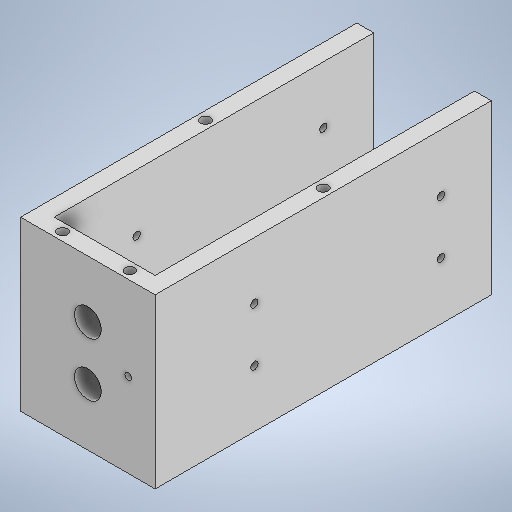
# Autodesk Inventor part: Handle_Main_Body
Saved by Autodesk Inventor 2026.2 (Build 302298010, 298A)
## iProperties
Created: 2026-04-30
Part Number: Handle_Main_Body
Material: Generic
Document SubType Name: Modeling
Designer: piete
Density: 1 g/cm^3
Appearance: Default
Author: piete
Autodesk Inventor part; units mm, degrees
ref_plane "YZ Plane" through (0, 0, 0) normal (1, 0, 0) x (0, 1, 0)
ref_plane "XY Plane" through (0, 0, 0) normal (0, 0, 1) x (1, 0, 0)
sketch "Sketch1" plane through (0, 0, 0) normal (0, 1, 0) x (-1, 0, 0)
  line L0 (20, 50) -> (-20, 50)
  line L1 (-20, 50) -> (-20, -50)
  line L2 (-20, -50) -> (20, -50)
  line L3 (20, -50) -> (20, 50)
  line L4 (15, 45) -> (-15, 45)
  line L5 (-15, 45) -> (-15, -45)
  line L6 (-15, -45) -> (15, -45)
  line L7 (15, -45) -> (15, 45)
  line L8 (15, -45) -> (15, -50)
  line L9 (-15, -45) -> (-15, -50)
  point P0 (0, 0)
  dimension "d0" = 40
  dimension "d1" = 100
  dimension "d2" = 20
  dimension "d3" = 50
  dimension "d4" = 5
  constraints: 20 end point, 4 parallel, 4 perpendicular, 2 point on line, 1 horizontal, 3 other
  measures "d0" distance of L2.end L1.end
  measures "d1" distance of L1.end L0.end
  measures "d2" distance from line of point (0, 0) L3
  measures "d3" distance from line of point (0, 0) L0
  measures "d4" distance between parallel lines of L3 L7
extrude "Extrusion1" add sketch "Sketch1" along normal blind 50 contours L3 L2 L8 L7 L4 L5 L9 L1 L0
sketch "Sketch2" plane through (-20, 0, 50) normal (0, 0, 1) x (1, 0, 0)
  circle A0 centre (20, 33) radius 4
  circle A1 centre (20, 17) radius 4
  circle A2 centre (32, 25) radius 1
  line L0 (0, 0) -> (40, 0) projected
  line L1 (40, 0) -> (40, 50) projected
  point P0 (20, 0)
  point P1 (20, 0)
  point P2 (20, 0)
  dimension "d7" = 8
  dimension "d8" = 8
  dimension "d9" = 2
  dimension "d10" = 0
  dimension "d11" = 0
  dimension "d12" = 8
  dimension "d13" = 25
  dimension "d14" = 16
  dimension "d15" = 8
  constraints: 3 centre point, 2 midpoint
  measures "d7" diameter of A0
  measures "d8" diameter of A1
  measures "d9" diameter of A2
  measures "d10" horizontal distance of point (20, 0) A0.centre
  measures "d11" horizontal distance of point (20, 0) A1.centre
  measures "d12" distance from line of L1 A2.centre
  measures "d13" distance from line of L0 A2.centre
  measures "d14" distance of A0.centre A1.centre
  measures "d15" vertical distance of A1.centre A2.centre
extrude "Extrusion2" cut sketch "Sketch2" against normal up to surface (5 mm away)
sketch "Sketch3" plane through (-20, 0, 50) normal (0, 0, 1) x (1, 0, 0)
  circle A0 centre (20, 33) radius 4 projected
  circle A1 centre (20, 33) radius 6
  circle A2 centre (20, 17) radius 4 projected
  circle A3 centre (20, 17) radius 6
  point P0 (20, 0)
  dimension "d18" = 12
  dimension "d19" = 12
  constraints: 2 centre point, 2 coincident
  measures "d18" diameter of A1
  measures "d19" diameter of A3
extrude "Extrusion3" add sketch "Sketch3" against normal blind 8
sketch "Sketch4" plane through (-15, 0, -50) normal (0, 0, -1) x (-1, 0, 0)
  circle A0 centre (2.5, 47.5) radius 1.5
  line L0 (5, 0) -> (5, 50) projected
  line L1 (0, 50) -> (5, 50) projected
  circle A1 centre (-32.5, 47.5) radius 1.5
  line L2 (-35, 50) -> (-30, 50) projected
  line L3 (-35, 0) -> (-35, 50) projected
  circle A2 centre (-32.5, 2.5) radius 1.5
  circle A3 centre (2.5, 2.5) radius 1.5
  line L4 (-35, 0) -> (-30, 0) projected
  line L5 (0, 0) -> (5, 0) projected
  point P0 (-15, 0)
  point P1 (-32.5, 50)
  dimension "d22" = 3
  dimension "d23" = 2.5
  dimension "d24" = 2.5
  dimension "d25" = 3
  dimension "d26" = 2.5
  dimension "d27" = 2.5
  dimension "d28" = 3
  dimension "d29" = 3
  dimension "d30" = 2.5
  dimension "d31" = 2.5
  dimension "d32" = 2.5
  dimension "d33" = 2.5
  constraints: 4 centre point, 1 midpoint
  measures "d22" diameter of A0
  measures "d23" distance from line of L0 A0.centre
  measures "d24" distance from line of L1 A0.centre
  measures "d25" diameter of A1
  measures "d26" distance of point (-32.5, 50) A1.centre
  measures "d27" distance from line of L3 A1.centre
  measures "d28" diameter of A2
  measures "d29" diameter of A3
  measures "d30" distance from line of L4 A2.centre
  measures "d31" distance from line of L3 A2.centre
  measures "d32" distance from line of L5 A3.centre
  measures "d33" distance from line of L0 A3.centre
extrude "Extrusion4" cut sketch "Sketch4" against normal blind 5
sketch "Sketch5" plane through (-20, 0, -50) normal (-1, 0, 0) x (0, 0, 1)
  circle A0 centre (15, 33) radius 1.1
  circle A1 centre (70.5, 33) radius 1.1
  circle A2 centre (15, 17) radius 1.1
  circle A3 centre (70.5, 17) radius 1.1
  line L0 (0, 0) -> (0, 50) projected
  line L1 (0, 0) -> (100, 0) projected
  point P0 (50, 0)
  dimension "d36" = 2.2
  dimension "d37" = 2.2
  dimension "d38" = 2.2
  dimension "d39" = 2.2
  dimension "d40" = 55.5
  dimension "d41" = 0
  dimension "d42" = 55.5
  dimension "d43" = 16
  dimension "d44" = 16
  dimension "d45" = 0
  dimension "d46" = 15
  dimension "d47" = 17
  constraints: 4 centre point
  measures "d36" diameter of A0
  measures "d37" diameter of A1
  measures "d38" diameter of A2
  measures "d39" diameter of A3
  measures "d40" distance of A1.centre A0.centre
  measures "d41" horizontal distance of A0.centre A2.centre
  measures "d42" distance of A3.centre A2.centre
  measures "d43" distance of A3.centre A1.centre
  measures "d44" distance of A2.centre A0.centre
  measures "d45" vertical distance of A3.centre A2.centre
  measures "d46" distance from line of L0 A2.centre
  measures "d47" distance from line of L1 A2.centre
extrude "Extrusion5" cut sketch "Sketch5" against normal through all
sketch "Sketch6" plane through (0, 50, 0) normal (0, 1, 0) x (1, 0, 0)
  circle A0 centre (10, -47.5) radius 1.5
  circle A1 centre (-10, -47.5) radius 1.5
  line L0 (-20, -50) -> (20, -50) projected
  circle A2 centre (17.5, 2.5) radius 1.5
  line L1 (20, -50) -> (20, 50) projected
  circle A3 centre (-17.5, 2.5) radius 1.5
  line L2 (-20, 50) -> (-20, -50) projected
  line L3 (20, 50) -> (15, 50) projected
  line L4 (-15, 50) -> (-20, 50) projected
  point P0 (0, 0)
  point P1 (0, -50)
  point P2 (0, -50)
  dimension "d50" = 3
  dimension "d51" = 3
  dimension "d52" = 2.5
  dimension "d53" = 2.5
  dimension "d54" = 10
  dimension "d55" = 10
  dimension "d56" = 3
  dimension "d57" = 2.5
  dimension "d58" = 3
  dimension "d59" = 2.5
  dimension "d60" = 47.5
  dimension "d61" = 47.5
  constraints: 4 centre point, 2 midpoint
  measures "d50" diameter of A0
  measures "d51" diameter of A1
  measures "d52" distance from line of L0 A1.centre
  measures "d53" distance from line of L0 A0.centre
  measures "d54" horizontal distance of point (0, -50) A0.centre
  measures "d55" horizontal distance of point (0, -50) A1.centre
  measures "d56" diameter of A2
  measures "d57" distance from line of L1 A2.centre
  measures "d58" diameter of A3
  measures "d59" distance from line of L2 A3.centre
  measures "d60" distance from line of L3 A2.centre
  measures "d61" distance from line of L4 A3.centre
extrude "Extrusion6" cut sketch "Sketch6" against normal blind 5
ref_plane "Work Plane1" through (0, 25, 0) normal (0, 1, 0) x (-1, 0, 0)
mirror "Mirror1" about plane through (0, 25, 0) normal (0, 1, 0) of "Extrusion6"
equation "\"d2\" = 0.5 * d0"
equation "\"d3\" = 0.5 * d1"
body "Solid1"
